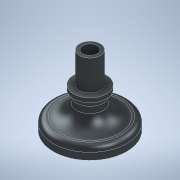
# Autodesk Inventor part: Bow Sling Rev B
Saved by Autodesk Inventor 2021 (Build 250183000, 183)
## iProperties
Created: 2021-08-19
Part Number: Bow Sling Rev B
Material: PC/ABS Plastic
Document SubType Name: Modeling
Designer: cmzgt
Density: 0.357273 g/cm^3
Appearance: Iron Gray
Author: cmzgt
## iProperties of the stored document _3DPrint.ipt
Created: 2021-08-19
Part Number: _3DPrint
Material: Generic
Document SubType Name: Modeling
Designer: cmzgt
Density: 1 g/cm^3
Appearance: Default
Author: cmzgt
Autodesk Inventor part; units mm, degrees
ref_plane "YZ Plane" through (0, 0, 0) normal (1, 0, 0) x (0, 1, 0)
ref_plane "XZ Plane" through (0, 0, 0) normal (0, 1, 0) x (-1, 0, 0)
ref_plane "XY Plane" through (0, 0, 0) normal (0, 0, 1) x (1, 0, 0)
sketch "Sketch1" plane through (0, 0, 0) normal (1, 0, 0) x (0, 1, 0)
  line L0 (0, 0) -> (0, -10.795)
  line L1 (0, -10.795) -> (2.54, -10.795)
  line L2 (0, 0) -> (12.7, 0)
  line L3 (2.54, -10.795) -> (2.54, -9.9414)
  line L4 (2.54, -9.9414) -> (2.54, -8.6714)
  line L5 (14.986, -3.937) -> (1.8235, -3.937) construction
  arc A0 (6.0461, -3.937) -> (2.54, -8.6714) centre (7.4896, -8.6714) ccw
  line L6 (9.398, -3.048) -> (9.398, -4.826)
  line L7 (6.0461, -3.937) -> (7.8921, -3.937)
  arc A1 (9.398, -4.826) -> (7.8921, -3.937) centre (7.8921, -5.6569) ccw
  line L8 (19.558, 0) -> (0, 0)
  line L9 (9.398, -3.048) -> (19.558, -3.048)
  line L10 (19.558, -3.048) -> (19.558, 0)
  dimension "d0" = 10.795
  dimension "d1" = 2.54
  dimension "d2" = 12.7
  dimension "d5" = 3.937
  dimension "d6" = 1.27
  dimension "d7" = 4.9496
  dimension "d18" = 4.826
  dimension "d19" = 1.7199
  dimension "d24" = 9.398
  dimension "d25" = 10.16
  dimension "d26" = 3.048
  dimension "d27" = 4.572
  dimension "d28" = 5.6234
  dimension "d29" = 17.7345
  constraints: 22 end point, 4 point on circle, 3 perpendicular, 3 point on line, 2 centre point, 2 horizontal, 2 tangent, 2 vertical, 1 collinear, 1 parallel
  measures "d0" distance of L0.start L0.end
  measures "d1" distance of L0.end L1.end
  measures "d2" distance of L0.start L2.end
  measures "d5" distance from line of L2 L5.start
  measures "d6" distance of L3.end L4.end
  measures "d7" radius of A0
  measures "d18" distance from line of L2 L6.end
  measures "d19" radius of A1
  measures "d24" distance between parallel lines of L0 L6
  measures "d25" distance of L6.start L9.end
  measures "d26" distance between parallel lines of L8 L9
  measures "d27" distance from line of L5.start L10
  measures "d28" distance from line of A0.centre L9
  measures "d29" distance from line of L5.end L10
revolve "Revolution1" add sketch "Sketch1" angle 360 about axis through (0, 0, 0) along (0, 1, 0)
sketch "Sketch2" plane through (0, 0, 0) normal (0, -1, 0) x (1, 0, 0)
  circle A0 centre (0, 0) radius 3.048 projected
  line L0 (4.95, -0.9536) -> (1.6491, -4.7636)
  line L1 (1.6491, -4.7636) -> (-3.3008, -3.81)
  line L2 (-3.3008, -3.81) -> (-4.95, 0.9536)
  line L3 (-4.95, 0.9536) -> (-1.6491, 4.7636)
  line L4 (-1.6491, 4.7636) -> (3.3008, 3.81)
  line L5 (3.3008, 3.81) -> (4.95, -0.9536)
  dimension "d11" = 8.7312
  dimension "d12" = 7.62
  constraints: 12 end point, 1 coincident, 13 other
  measures "d11" distance between parallel lines of L3 L0
  measures "d12" vertical distance of L1.end L4.end
extrude "Extrusion1" cut sketch "Sketch2" against normal blind 3.302 contours A0 | L0 L1 L2 L3 L4 L5
sketch "Sketch3" plane through (0, 3.302, 0) normal (0, -1, 0) x (1, 0, 0)
  circle A0 centre (0, 0) radius 2.0892
  dimension "d15" = 4.1783
  constraints: 1 centre point, 1 coincident
  measures "d15" diameter of A0
extrude "Extrusion2" cut sketch "Sketch3" against normal up to surface (16.256 mm away)
sketch "Sketch5" plane through (0, 9.398, 0) normal (0, 1, 0) x (1, 0, 0)
  circle A0 centre (0, 0) radius 4.826 projected
  circle A1 centre (0, 0) radius 3.048 projected
extrude "Extrusion5" add sketch "Sketch5" along normal blind 1.27
sketch "Sketch6" plane through (0, 0, 0) normal (0, -1, 0) x (1, 0, 0)
  circle A0 centre (0, 0) radius 10.795 projected
  line L0 (3.3008, 3.81) -> (4.95, -0.9536) projected
  line L1 (4.95, -0.9536) -> (1.6491, -4.7636) projected
  line L2 (1.6491, -4.7636) -> (-3.3008, -3.81) projected
  line L3 (-3.3008, -3.81) -> (-4.95, 0.9536) projected
  line L4 (-4.95, 0.9536) -> (-1.6491, 4.7636) projected
  line L5 (-1.6491, 4.7636) -> (3.3008, 3.81) projected
extrude "Extrusion6" add sketch "Sketch6" along normal blind 1.016
fillet "Fillet1" radius 1.524 1 edges at (0, 2.54, 10.795)
body "Solid1"
